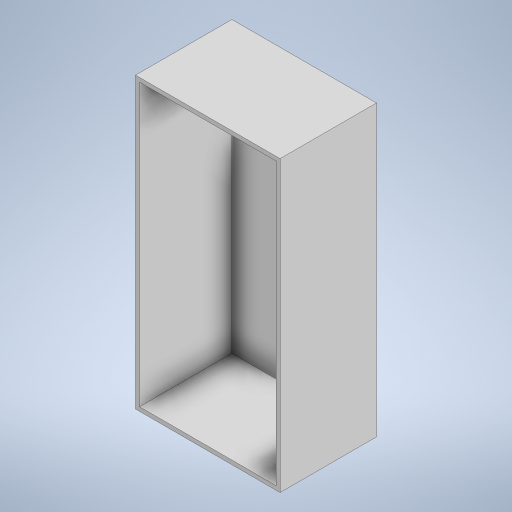
# Autodesk Inventor part: grey cabinet
Saved by Autodesk Inventor 2023 (Build 270158000, 158)
## iProperties
Created: 2022-11-15
Part Number: grey cabinet
Material: Generic
Document SubType Name: Modeling
Designer: 4026 User
Density: 1 g/cm^3
Appearance: Default
Author: 4026 User
Autodesk Inventor part; units mm, degrees
ref_plane "YZ Plane" through (0, 0, 0) normal (1, 0, 0) x (0, 1, 0)
ref_plane "XZ Plane" through (0, 0, 0) normal (0, 1, 0) x (-1, 0, 0)
ref_plane "XY Plane" through (0, 0, 0) normal (0, 0, 1) x (1, 0, 0)
sketch "grey cabinet" plane through (0, 0, 0) normal (0, 1, 0) x (-1, 0, 0)
  line L0 (914.4, 609.6) -> (0, 609.6)
  line L1 (0, 609.6) -> (0, 0)
  line L2 (0, 0) -> (914.4, 0)
  line L3 (914.4, 0) -> (914.4, 609.6)
  dimension "d0" = 914.4
  dimension "d1" = 609.6
  constraints: 8 end point, 2 parallel, 1 coincident, 1 horizontal, 1 perpendicular
  measures "d0" distance of L0.start L0.end
  measures "d1" distance of L2.end L0.start
extrude "grey cabinet2" add sketch "grey cabinet" along normal blind 1828.8
shell "Shell1" thickness 25.4 removed faces 1 at (-609.6, 609.6, 609.6)
